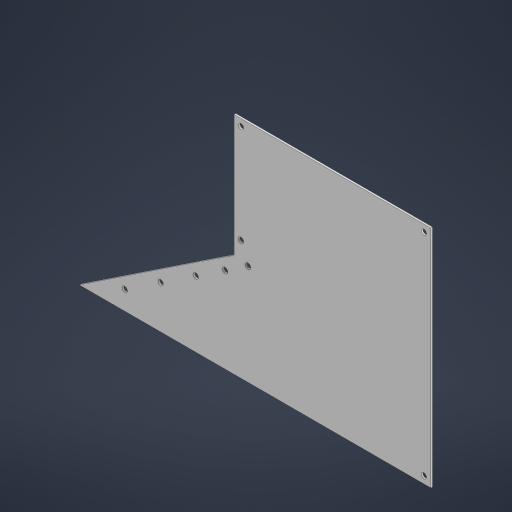
# Autodesk Inventor part: intakeabs2
Saved by Autodesk Inventor 2023 (Build 270158000, 158)
## iProperties
Created: 2023-02-28
Part Number: intakeabs2
Material: Generic
Document SubType Name: Modeling
Designer: Windows Macbook
Density: 1 g/cm^3
Appearance: Default
Author: Windows Macbook
Autodesk Inventor part; units mm, degrees
ref_plane "YZ Plane" through (0, 0, 0) normal (1, 0, 0) x (0, 1, 0)
ref_plane "XZ Plane" through (0, 0, 0) normal (0, 1, 0) x (-1, 0, 0)
ref_plane "XY Plane" through (0, 0, 0) normal (0, 0, 1) x (1, 0, 0)
sketch "Sketch1" plane through (0, 0, 0) normal (0, 0, 1) x (1, 0, 0)
  line L0 (0, 203.2) -> (-152.4, 203.2)
  line L1 (0, 0) -> (-304.8, 0)
  line L2 (-304.8, 0) -> (-165.1, 93.1333)
  line L3 (-152.4, 203.2) -> (-165.1, 203.2)
  line L4 (-165.1, 203.2) -> (-165.1, 93.1333)
  line L5 (0, 203.2) -> (12.7, 203.2)
  line L6 (12.7, 203.2) -> (12.7, 0)
  line L7 (12.7, 0) -> (0, 0)
  dimension "d0" = 203.2
  dimension "d1" = 152.4
  dimension "d2" = 304.8
  dimension "d5" = 12.7
  dimension "d6" = 12.7
  constraints: 16 end point, 3 horizontal, 3 perpendicular, 2 point on line
  measures "d0" distance of L1.start L0.start
  measures "d1" distance of L0.start L0.end
  measures "d2" distance of L1.start L1.end
  measures "d5" distance of L0.end L3.end
  measures "d6" distance of L5.start L5.end
extrude "Extrusion1" add sketch "Sketch1" along normal blind 1.5875
sketch "Sketch2" plane through (0, 0, 1.5875) normal (0, 0, 1) x (1, 0, 0)
  line L0 (12.7, 203.2) -> (-165.1, 203.2) projected
  line L1 (-165.1, 203.2) -> (-158.75, 203.2)
  line L2 (-304.8, 0) -> (12.7, 0) projected
  line L3 (12.7, 203.2) -> (6.35, 203.2)
  line L4 (-302.2289, 0) -> (-289.5289, 0)
  line L5 (-165.1, 203.2) -> (-152.4, 203.2)
  line L6 (-158.75, 203.2) -> (-158.75, 196.85)
  line L7 (-158.75, 101.6) -> (-158.75, 107.95)
  line L8 (6.35, 203.2) -> (6.35, 196.85)
  line L9 (6.35, 0) -> (6.35, 6.35)
  point P0 (0, 0)
  point P1 (-263.7214, 17.1277)
  point P2 (-231.3298, 38.625)
  point P3 (-199.5848, 59.6931)
  point P4 (-173.1307, 77.2499)
  point P5 (-152.4, 91.0082)
  dimension "d7" = 6.35
  dimension "d8" = 6.35
  dimension "d14" = 12.7
  dimension "d15" = 6.35
  dimension "d16" = 101.6
  dimension "d17" = 6.35
  dimension "d18" = 6.35
  dimension "d19" = 6.35
  constraints: 16 end point, 5 point on line, 4 coincident
  measures "d7" distance of L0.end L1.end
  measures "d8" distance of L0.start L3.end
  measures "d14" distance of L0.end L5.end
  measures "d15" distance of L1.end L6.end
  measures "d16" distance of L1.end L7.start
  measures "d17" distance of L7.start L7.end
  measures "d18" distance of L3.end L8.end
  measures "d19" distance of L9.start L9.end
hole "Hole1" at (-263.7214, 17.1277, 1.5875) at (-231.3298, 38.625, 1.5875) at (-199.5848, 59.6931, 1.5875) at (-173.1307, 77.2499, 1.5875) at (-152.4, 91.0082, 1.5875) at (-158.75, 107.95, 1.5875) at (-158.75, 196.85, 1.5875) at (6.35, 6.35, 1.5875) at (6.35, 196.85, 1.5875) direction (0, 0, -1) diameter 4.7625 end through all
body "Solid1"
